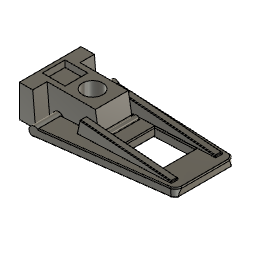
FoldingFoot-small (Autodesk Fusion 360 design; units mm, degrees)
Autodesk Fusion 360 part; units mm, degrees
note: some values were not read from the file. Chosen so that the rebuilt part matches the saved one: which bodies a step acts on; which face or edge a step refers to; the sign of a taper; which pieces of a blend or face edit are solid. Set by a fixed rule: which sketch regions a step uses.
sketch "Sketch1" plane through (0, 0, 0) normal (0, 0, 1) x (1, 0, 0)
  line L0 (0, 0) -> (40.373044, 3.561977)
  line L1 (0, 12.73) -> (61.000001, 12.73) construction
  arc A0 (40.373044, 3.561977) -> (42, 5.83) centre (39.501125, 5.905) ccw
  line L2 (42, 5.83) -> (42, 12.73)
  line L3 (11.3, 6.92) -> (39.3, 6.92)
  line L4 (39.3, 6.92) -> (39.3, 4.82)
  line L5 (39.3, 4.82) -> (11.3, 4.82)
  line L6 (11.3, 4.82) -> (11.3, 6.92)
  line L7 (33.4, 12.73) -> (33.4, 7.34)
  line L8 (33.4, 7.34) -> (20.8, 7.34)
  line L9 (20.8, 7.34) -> (20.8, 12.73)
  line L10 (1.5, 12.740731) -> (1.5, 7.34)
  line L11 (1.5, 7.34) -> (15.8, 7.34)
  line L12 (15.8, 7.34) -> (15.8, 12.740731)
  line L13 (0, 12.73) -> (42, 12.73)
  line L14 (0, 12.73) -> (0, 0)
  line L15 (0, 18.19) -> (42, 18.19)
  line L16 (1.5, 7.34) -> (0, 7.34)
  line L17 (1.5, 7.34) -> (1.5, 0.13234)
  line L18 (0, 12.73) -> (0, 25.46)
  line L19 (0, 25.46) -> (40.373044, 21.898023)
  line L20 (1.5, 18.12) -> (1.5, 25.32766)
  line L21 (39.3, 20.64) -> (11.3, 20.64)
  line L22 (11.3, 20.64) -> (11.3, 18.54)
  line L23 (11.3, 18.54) -> (39.3, 18.54)
  line L24 (39.3, 18.54) -> (39.3, 20.64)
  arc A1 (42, 19.63) -> (40.373044, 21.898023) centre (39.501125, 19.555) ccw
  line L25 (42, 19.63) -> (42, 12.73)
  line L26 (1.5, 12.719269) -> (1.5, 18.12)
  line L27 (1.5, 18.12) -> (15.8, 18.12)
  line L28 (15.8, 18.12) -> (15.8, 12.719269)
  line L29 (20.8, 18.12) -> (20.8, 12.73)
  line L30 (33.4, 12.73) -> (33.4, 18.12)
  line L31 (33.4, 18.12) -> (20.8, 18.12)
  dimension "d2" = 2.1
  dimension "d37" = 11.3
  dimension "d96" = 1.5
  dimension "d121" = 42
  dimension "d125" = 14.3
  dimension "d157" = 28
  dimension "d159" = 5
  dimension "d160" = 12.6
  dimension "d161" = 12.73
  dimension "d162" = 5.39
  dimension "d164" = 2.5
  dimension "d165" = 6.825
  dimension "d169" = 6.9
  dimension "d170" = 8.6
  dimension "d171" = 5.81
  constraint coincident L0.start L14.end
  constraint horizontal L1
  constraint coincident L1 L2.end
  constraint perpendicular L1 L2
  constraint horizontal L3
  constraint vertical L4
  constraint horizontal L5
  constraint vertical L6
  constraint vertical L7
  constraint horizontal L8
  constraint vertical L9
  constraint coincident L1 L9.end
  constraint vertical L10
  constraint horizontal L11
  constraint vertical L12
  constraint collinear L8 L11
  constraint parallel L10 L14
  constraint coincident L14 L16.end
  constraint perpendicular L14 L16
  constraint perpendicular L16 L17
  constraint collinear L10 L17
  constraint symmetric L0.start L1 L18.end
  constraint symmetric L13.start L1 L14.start
  constraint symmetric L1 A0.end A1.start
  constraint symmetric L1 A0 A1
  constraint symmetric L1 L2.end L13.end
  constraint symmetric L1 L3.start L22.end
  constraint symmetric L1 L3.end L23.end
  constraint symmetric L1 L4.end L21.start
  constraint symmetric L1 L5.end L21.end
  constraint symmetric L1 L9.end L29.end
  constraint symmetric L1 L7.start L30.start
  constraint symmetric L1 L7.end L30.end
  constraint symmetric L1 L8.end L29.start
  constraint symmetric L1 L10.end L20.start
  constraint symmetric L1 L11.end L27.end
  constraint symmetric L1 L0.start L18.end
  measures "d2" distance of L3 L5
  measures "d37" distance of L6 L14
  measures "d96" distance of L14 L17
  measures "d121" distance of L15.start L15.end
  measures "d125" distance of L10.end L11.end
  measures "d157" distance of L4.end L5.end
  measures "d159" distance of L9 L12
  measures "d160" distance of L7 L9
  measures "d161" distance of L1.start L0.start
  measures "d162" distance of L11 L13
  measures "d164" radius of A0
  measures "d169" distance of A0.end L2.end
  measures "d170" distance of L2 L7
  measures "d171" distance of L1 L3
extrude "Extrude1" add sketch "Sketch1" along normal blind 2.6 contours L0 A0 L2 L7 L8 L9 L11 L12 L13 L17 L28 | L12 L13 L15 L20 L25 L27 L28 L29 L30 L31 | L15 L19 L20 A1 L25 | L3 L4 L5 L6 | L21 L22 L23 L24 picked at (4.766667, 4.097447) picked at (39.133333, 16.346667) picked at (4.766667, 21.385887) picked at (29.966667, 5.52) picked at (29.966667, 19.24) makes body 1
extrude "Extrude2" add sketch "Sketch1" along normal blind 6.6 contours L3 L4 L5 L6 | L21 L22 L23 L24 picked at (29.966667, 5.52) picked at (29.966667, 19.24) bodies 1
sketch "Sketch1 (2)" plane through (0, 0, 0) normal (0, 0, 1) x (1, 0, 0) in component "geraetefuss-halter v4"
  line L0 (0.051446, -5.09) -> (15.151446, -5.09)
  line L1 (15.151446, -5.09) -> (15.151446, -9.53)
  line L2 (15.151446, -9.53) -> (20.151446, -9.53)
  line L3 (20.151446, -9.53) -> (20.151446, 0)
  line L4 (0.051446, 0) -> (0.051446, -5.09)
  circle A0 centre (7.051446, 0) radius 3.15
  circle A1 centre (7.051446, 0) radius 1.7
  line L5 (19.051446, -3.5) -> (12.051446, -3.5)
  line L6 (12.051446, -3.5) -> (12.051446, 3.5)
  line L7 (12.051446, 3.5) -> (19.051446, 3.5)
  line L8 (19.051446, 3.5) -> (19.051446, -3.5)
  line L9 (19.051446, -3.5) -> (12.051446, 3.5) construction
  line L10 (12.051446, -3.5) -> (19.051446, 3.5) construction
  line L11 (0.051446, 0) -> (20.151446, 0) construction
  line L12 (0.051446, 0) -> (0.051446, 5.09)
  line L13 (0.051446, 5.09) -> (15.151446, 5.09)
  line L14 (15.151446, 5.09) -> (15.151446, 9.53)
  line L15 (15.151446, 9.53) -> (20.151446, 9.53)
  line L16 (20.151446, 9.53) -> (20.151446, 0)
  line L17 (1.75, 0) -> (22.5, 0)
  point P0 (15.551446, 0)
  dimension "d1" = 6.3
  dimension "d2_1" = 7
  dimension "d3_1" = 3.4
  dimension "d5_1" = 15.1
  dimension "d6_1" = 5
  dimension "d7_1" = 4.44
  dimension "d18_1" = 7
  dimension "d19_1" = 7
  dimension "d20_1" = 12
  dimension "d82" = 5.09
  dimension "d174" = 5.09
  dimension "d175" = 5.09
  constraint perpendicular L0 L1
  constraint perpendicular L1 L2
  constraint perpendicular L0 L3
  constraint perpendicular L0 L4
  constraint concentric A0 A1
  constraint horizontal L5
  constraint perpendicular L5 L6
  constraint parallel L5 L7
  constraint parallel L6 L8
  constraint perpendicular L3 L11
  constraint collinear L11 L17
  measures "d1" diameter of A0
  measures "d3_1" diameter of A1
  measures "d20_1" distance of L4 L6
extrude "Extrude8" add sketch "Sketch1 (2)" along normal blind 5 separate body contours A0 A1 L17 | A0 A1 L17 picked at (4.402837, 0.240952) picked at (9.700056, -0.240952) makes body 2 in component "geraetefuss-halter v4"
extrude "Extrude7" add sketch "Sketch1 (2)" along normal blind 8 separate body contours L5 L6 L8 L17 | L6 L7 L8 L17 picked at (14.38478, -1.166667) picked at (14.38478, 2.333333) makes body 3 in component "geraetefuss-halter v4"
extrude "Extrude6" add sketch "Sketch1 (2)" along normal blind 10 separate body contours L0 L1 L2 L3 L4 L12 L13 L14 L15 L16 picked at (18.118113, 6.04) makes body 4 in component "geraetefuss-halter v4"
sketch "Sketch4" plane through (0, -5.09, 0) normal (0, -1, 0) x (1, 0, 0) in component "geraetefuss-halter v4"
  line L0 (0, 0) -> (17, 0)
  line L1 (17, 10) -> (0, 10)
  line L2 (0, 10) -> (0, 0)
  line L3 (0, 5) -> (15.151446, 5) construction
  circle A0 centre (12.501446, 2.1) radius 1.65
  line L4 (10.851446, 2.1) -> (10.851446, 0)
  line L5 (14.151446, 2.1) -> (14.151446, 0)
  line L6 (0.051446, 0) -> (15.151446, 0)
  line L7 (15.151446, 0) -> (15.151446, 10)
  line L8 (15.151446, 10) -> (0.051446, 10)
  line L9 (0.051446, 10) -> (0.051446, 0)
  dimension "d13_1" = 3.3
  dimension "d53" = 2.1
  dimension "d128" = 1
  constraint midpoint L2 L3.start
  constraint perpendicular L0 L4
  constraint perpendicular L0 L5
  constraint tangent A0 L4
  constraint tangent A0 L5
  constraint horizontal L3
  measures "d13_1" diameter of A0
extrude "Extrude9" cut sketch "Sketch4" against normal up to surface (10.18 mm away) contours L0 A0 L4 L5 L6 | A0 picked at (12.542548, 0.151538) picked at (12.047015, 1.790174) bodies 4 3 in component "geraetefuss-halter v4"
draft "Draft1" angle -7 neutral plane through (11.3, 20.64, 0) pull (-1, 0, 0) 2 faces at (29.966667, 19.24, 6.6) (29.966667, 5.52, 6.6) on bodies 1
copy_body "Body->Comp1" bodies 1 removing the originals makes body 5 in component "Fuss"
move_body "Move1" bodies 5 to x (1, 0, 0) y (0, 1, 0) z (0, 0, 1) at (19, 0, 0) in component "Fuss"
combine "Combine2" operation add target body 4 tool bodies 3 in component "geraetefuss-halter v4"
combine "Combine3" operation add target body 4 tool bodies 2 in component "geraetefuss-halter v4"
draft "Draft3" angle -10 neutral plane through (19, 0, 2.6) pull (0, 0, 1) 1 faces at (61, 10.43, 0.866667) on bodies 5 in component "Fuss"
move_body "Move5" bodies 4 to x (-1, 0, 0) y (0, -1, 0) z (0, 0, 1) at (11.102893, -7.117, 0) in component "geraetefuss-halter v4"
draft "Draft7" angle -5 neutral plane through (11.102893, -7.117, 0) pull (0, 0, -1) 1 faces at (-4.048554, -13.687, 3.333333) on bodies 4 in component "geraetefuss-halter v4"
draft "Draft8" angle 5 neutral plane through (11.102893, -7.117, 0) pull (0, 0, 1) 1 faces at (-4.048554, -0.547, 3.333333) on bodies 4 in component "geraetefuss-halter v4"
sketch "Sketch19" plane through (0, 7.34, 0) normal (0, 1, 0) x (-1, 0, 0)
  line L0 (-34.8, 0) -> (-20.5, 0)
  line L1 (-20.5, 0) -> (-20.5, 2.6)
  line L2 (-20.5, 2.6) -> (-34.8, 2.6)
  line L3 (-34.8, 2.6) -> (-34.8, 0)
  circle A0 centre (-20.542806, 1.5) radius 1.5
  line L4 (-20.5, 0) -> (-59.373044, 0)
  dimension "d97" = 3
  constraint tangent A0 L4
  measures "d97" diameter of A0
extrude "Extrude1'" add sketch "Sketch19" along normal up to surface and the other way up to surface contours L1 L2 A0 | L1 L2 A0 picked at (-20.571137, 0.870114) picked at (-20.430301, 0.873768) end surface through (20.5, 25.32766, 0) normal (0.08788523, 0.99613061, 0) offset 0 second end surface through (20.5, 0.13234, 0) normal (-0.08788523, 0.99613061, 0) offset 0 bodies 5 in component "Fuss"
draft "Draft4" angle 15 neutral plane through (19.084228, 0, 7.977124) pull (0.121869, 0, 0.992546) 1 faces at (30.3, 6.22, 5.266667) on bodies 5 in component "Fuss"
draft "Draft5" angle 15 neutral plane through (19.084228, 0, 7.977124) pull (0.121869, 0, 0.992546) 1 faces at (30.3, 19.94, 3.933333) on bodies 5 in component "Fuss"
fillet "Fillet1" radius 0.3 9 edges at (39.936522, 1.847158, 0) (60.025021, 3.923147, 0) (60.54155, 12.73, 0) (39.936522, 23.612842, 0) (40.467827, 1.894034, 2.6) (61, 12.73, 2.6) (40.467827, 23.565966, 2.6) (60.532515, 21.012208, 2.6) (60.532515, 4.447792, 2.6) on bodies 5 in component "Fuss"
fillet "Fillet2" radius 0.3 7 edges at (46.1, 7.34, 0) (52.4, 12.73, 0) (39.8, 12.73, 0) (52.4, 12.73, 2.6) (46.1, 7.34, 2.6) (39.8, 12.73, 2.6) (46.1, 18.12, 2.6) on bodies 5 in component "Fuss"
fillet "Fillet3" radius 0.2 6 edges at (44.3, 4.82, 4.881016) (44.3, 6.92, 4.881016) (44.3, 20.64, 4.881016) (44.3, 18.54, 4.881016) (58.3, 5.87, 3.162032) (58.3, 19.59, 3.162032) on bodies 5 in component "Fuss"
sketch "Sketch20" plane through (11.051446, 0, 0) normal (1, 0, 0) x (0, 1, 0)
  line L0 (-4.207, 10) -> (5.973, 10)
  line L1 (5.973, 10) -> (5.973, 20)
  line L2 (5.973, 20) -> (-4.207, 20)
  line L3 (-4.207, 20) -> (-4.207, 10)
  line L4 (-6.5255, 14) -> (8.2915, 14)
  dimension "d148" = 4
  measures "d148" distance of L0 L4
split "Split2" by curves path "Sketch20" along L4 path seen with x (1, 0, 0) y (0, 1, 0) z (0, 0, 1) at (0, -8, -10) bodies 4 makes body 6 at (-7.381887, -8.813667, 0) in component "geraetefuss-halter v4"
draft "Draft10" angle -10 neutral plane through (-988.948554, -14.5255, 4) pull (0, 0, -1) 1 faces at (11.051446, -8.813667, 6) on bodies 4 in component "geraetefuss-halter v4"
sketch "Sketch22" plane through (11.051446, 0, 0) normal (1, 0, 0) x (0, 1, 0)
  line L0 (5.973, 14) -> (-4.207, 14)
  line L1 (-4.207, 14) -> (-4.207, 10)
  line L2 (-4.207, 10) -> (5.973, 10)
  line L3 (5.973, 10) -> (5.973, 14)
  line L4 (-4.207, 10.6) -> (5.973, 10.6)
  dimension "d147" = 0.6
  constraint coincident L1 L4.start
  constraint coincident L3 L4.end
  constraint perpendicular L3 L4
  measures "d147" distance of L2 L4
extrude "Extrude11" add sketch "Sketch22" along normal blind 1.5 contours L1 L2 L3 L4 picked at (-0.813667, 10.4) sketch seen with x (1, 0, 0) y (0, 1, 0) z (0, 0, 1) at (0, -8, -10) bodies 6 in component "geraetefuss-halter v4"
sketch "Sketch23" plane through (0, 0, 10.6) normal (0, 0, 1) x (-1, 0, 0)
  line L0 (-11.051446, -5.973) -> (-11.051446, 4.207)
  line L1 (-11.051446, 4.207) -> (-12.551446, 4.207)
  line L2 (-12.551446, 4.207) -> (-12.551446, -5.973)
  line L3 (-12.551446, -5.973) -> (-11.051446, -5.973)
  line L4 (-12.251446, -5.973) -> (-12.251446, 4.207)
  dimension "d149" = 0.3
  measures "d149" distance of L2 L4
sketch "Sketch25" plane through (0, 5.973, 0) normal (0, 1, 0) x (-1, 0, 0)
  line L0 (4.398508, 14) -> (-11.051446, 14)
  line L1 (-11.051446, 14) -> (-11.051446, 10.6)
  line L2 (-11.051446, 10.6) -> (-12.551446, 10.6)
  line L3 (-12.551446, 10.6) -> (-12.551446, 10)
  line L4 (-12.551446, 10) -> (-0.251446, 10)
  line L5 (-0.251446, 10) -> (-0.251446, 12.1)
  arc A0 (3.048554, 12.1) -> (-0.251446, 12.1) centre (1.398554, 12.1) ccw
  line L6 (3.048554, 12.1) -> (3.048554, 10)
  line L7 (4.048554, 10) -> (4.398508, 14)
  spline S0 degree 5 poles (-12, 14) (-11.99718, 14.034418) (-11.994394, 14.101383) (-11.998775, 14.196219) (-12.021811, 14.311397) (-12.079229, 14.43618) (-12.164473, 14.541019) (-12.275333, 14.624768) (-12.407613, 14.685876) (-12.554255, 14.72231) (-12.706238, 14.732054) (-12.853812, 14.713732) (-12.987649, 14.667264) (-13.099908, 14.594448) (-13.185675, 14.499927) (-13.242991, 14.390814) (-13.271833, 14.275335) (-13.273435, 14.161752) (-13.249567, 14.057283) (-13.20178, 13.966757) (-13.131212, 13.892772) (-13.057166, 13.847731) (-12.991934, 13.822005) (-12.944154, 13.80842) (-12.919191, 13.802519) knots 0 0 0 0 0 0 0.05 0.1 0.15 0.2 0.25 0.3 0.35 0.4 0.45 0.5 0.55 0.6 0.65 0.7 0.75 0.8 0.85 0.9 0.95 1 1 1 1 1 1
  spline S1 degree 2 poles (-12.919191, 13.802519) (-12.583435, 11.821586) (-12.551446, 10.6) knots 0 0 0 0.32277411 0.32277411 0.32277411 weights 1 3 1
  spline S2 degree 2 poles (-12, 14) (-11.82976, 11.887123) (-11.801446, 10.6) knots 0 0 0 0.34065405 0.34065405 0.34065405 weights 1 3 1
  line L8 (3.048554, 10) -> (4.048554, 10)
  point P0 (-12.303953, 14.632375)
  point P1 (-13.033654, 14.632375)
  point P2 (-13.262579, 14.1316)
extrude "Extrude12" add sketch "Sketch25" against normal up to surface (10.18 mm away) contours L2 S0 S1 S2 picked at (-12.513532, 13.239675) sketch seen with x (1, 0, 0) y (0, 1, 0) z (0, 0, 1) at (0, -8, -10) bodies 6 in component "geraetefuss-halter v4"
combine "Combine4" operation add target body 4 tool bodies 6 in component "geraetefuss-halter v4"
fillet "Fillet4" radius 0.5 2 edges at (34.8, 12.73, 0) (34.8, 12.73, 2.6) on bodies 5 in component "Fuss"
component "geraetefuss-halter v4" placed x (1, 0, 0) y (0, 1, 0) z (0, 0, 1) at (0, 8, 10)
component "Fuss" placed x (1, 0, 0) y (0, 1, 0) z (0, 0, 1) at (-21.94136, -11.847, 10.6)
equation "d2 = FussStegBreite"
equation "d3 = FussHoehe"
equation "d5 = FussStegHoehe + FussHoehe"
equation "d1 = 6.0 mm + PrintMargin"
equation "d3_1 = 3.1 mm + PrintMargin"
equation "d5_1 = FussInnenAusspLaenge + FussAchsen_d / 2 + 1 mm"
equation "d6_1 = HalterTLaenge"
equation "d13_1 = FussAchsen_d + PrintMargin"
equation "FussAchsen_d = 3.0 mm" comment "Durchmesser Fuss-Achse"
equation "FussInnenAusspBreite = 10.78 mm" comment "v"
equation "HalterHoehe = 10 mm"
equation "EntfSteg_Achse = HalterHoehe"
equation "d37 = HalterHoehe - FussAchsen_d / 2 + 2.5 mm + PrintMargin"
equation "HalterTLaenge = 5 mm" comment "laenge T-stueck Halter oberkante"
equation "HalterTBreite = 24 mm" comment "Breite T-stueck Halter oberkante"
equation "FussStegHoehe = HalterTLaenge - 1 mm"
equation "FussInnenAusspLaenge = 12.6 mm" comment "v Abstand Innenkante Aussp. - Achsenmitte"
equation "d53 = FussAchsen_d / 2 + 0.6 mm"
equation "PrintMargin = 0.3 mm"
equation "d82 = FussInnenAusspBreite / 2 - PrintMargin"
equation "d83 = HalterHoehe"
equation "d85 = HalterHoehe - 2 mm"
equation "d87 = HalterHoehe - 5 mm"
equation "FussHoehe = 2.6 mm"
equation "d96 = FussAchsen_d / 2"
equation "d97 = FussAchsen_d"
equation "d121 = FussLaenge"
equation "FussLaenge = 42 mm" comment "v"
equation "d125 = FussInnenAusspLaenge + 1.7 mm"
equation "d157 = FussStegLaenge"
equation "FussStegLaenge = 28 mm" comment "v"
equation "d162 = FussInnenAusspBreite / 2"
equation "FussStegBreite = 2.1 mm" comment "v Breite der beiden Stege"
equation "d174 = FussInnenAusspBreite / 2 - PrintMargin"
equation "d175 = FussInnenAusspBreite / 2 - PrintMargin"
named bodies: "Fuss", "Fuss-halter", "Fuss-halter (1)"
